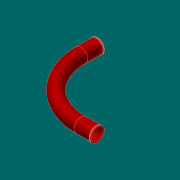
# Autodesk Inventor part: A1-19027-100-xx HCWI elbow
Saved by Autodesk Inventor 2017.3 (Build 213256000, 256)
## iProperties
Created: 2019-06-26
Part Number: A1-19027-100-xx HCWI elbow
Material: Iron, HCWI
Document SubType Name: Modeling
Designer: Graeme_Van_Dongen
Density: 7.33517 g/cm^3
Appearance: Iron Gray(1)
Mass: 7.05374e+06 g
Surface Area: 379961 cm^2
Volume: 961633 cm^3
Author: Graeme_Van_Dongen
Autodesk Inventor part; units mm, degrees
ref_plane "YZ Plane" through (0, 0, 0) normal (1, 0, 0) x (0, 1, 0)
ref_plane "XZ Plane" through (0, 0, 0) normal (0, 1, 0) x (-1, 0, 0)
ref_plane "XY Plane" through (0, 0, 0) normal (0, 0, 1) x (1, 0, 0)
sketch "Sketch1" plane through (0, 0, 0) normal (0, 0, 1) x (1, 0, 0)
  circle A0 centre (-3657.6, 0) radius 361.95
  circle A1 centre (-3657.6, 0) radius 412.75
  line L0 (0, -577.85) -> (0, 577.85) projected
  point P0 (0, 0)
  dimension "d0" = 723.9
  dimension "d1" = 825.5
  dimension "d2" = 3657.6
  constraints: 2 centre point, 1 coincident, 1 horizontal alignment
  measures "d0" diameter of A0
  measures "d1" diameter of A1
  measures "d2" distance of point (0, 0) A0.centre
revolve "Revolution1" add sketch "Sketch1" angle 90 about axis through (0, -10, 0) along (0, 1, 0)
sketch "Sketch2" plane through (-3657.6, 0, 0) normal (0, 0, -1) x (-1, 0, 0)
  circle A0 centre (0, 0) radius 361.95 projected
  circle A1 centre (0, 0) radius 412.75 projected
  point P0 (-3657.6, 0)
extrude "Extrusion1" add sketch "Sketch2" along normal blind 983.4
sketch "Sketch3" plane through (0, 0, 3657.6) normal (1, 0, 0) x (0, 0, -1)
  circle A0 centre (0, 0) radius 361.95 projected
  circle A1 centre (0, 0) radius 412.75 projected
  point P0 (3657.6, 0)
extrude "Extrusion2" add sketch "Sketch3" along normal blind 983.4
sketch "Sketch8" plane through (-3657.6, 0, -983.4) normal (0, 0, -1) x (-1, 0, 0)
  circle A0 centre (0, 0) radius 412.75 projected
  circle A1 centre (0, 0) radius 438.15
  point P0 (-3657.6, 0)
  dimension "d25" = 876.3
  constraints: 1 centre point, 1 coincident
  measures "d25" diameter of A1
extrude "Extrusion7" add sketch "Sketch8" against normal blind 50.8
sketch "Sketch9" plane through (983.4, 0, 3657.6) normal (1, 0, 0) x (0, 0, -1)
  circle A0 centre (0, 0) radius 412.75 projected
  circle A1 centre (0, 0) radius 361.95 projected
  circle A2 centre (0, 0) radius 438.15
  point P0 (3657.6, 0)
  dimension "d28" = 876.3
  constraints: 1 centre point, 1 coincident
  measures "d28" diameter of A2
extrude "Extrusion8" add sketch "Sketch9" against normal blind 50.8 contours A2
chamfer "Chamfer2" distance 25.4 angle 45 2 edges at (932.6, 0, 4070.35) (-3244.85, 0, -932.6)
sketch "Sketch5" plane through (-3657.6, 0, -983.4) normal (0, 0, -1) x (-1, 0, 0)
  circle A0 centre (0, 0) radius 434.721
  circle A1 centre (0, 0) radius 438.15 projected
  point P0 (-4064, 0)
  dimension "d11" = 869.442
  constraints: 1 centre point, 1 coincident
  measures "d11" diameter of A0
extrude "Extrusion4" cut sketch "Sketch5" against normal blind 25.4
sketch "Sketch7" plane through (983.4, 0, 3657.6) normal (1, 0, 0) x (0, 0, -1)
  circle A0 centre (0, 0) radius 434.721
  circle A1 centre (0, 0) radius 438.15 projected
  point P0 (4064, 0)
  dimension "d17" = 869.442
  constraints: 2 coincident, 1 centre point
  measures "d17" diameter of A0
extrude "Extrusion6" cut sketch "Sketch7" against normal blind 25.4
fillet "Fillet2" radius 0.7937 2 edges at (958, 0, 4092.321) (-3222.879, 0, -958)
equation "\"d6\" = d4"
equation "\"d28\" = d25"
equation "\"d29\" = d26"
equation "\"d31\" = -0.5 * d1 + 0.5 * d25"
equation "\"d17\" = d11"
equation "\"d18\" = d12"
equation "\"d4\" = 983.4"
equation "\"d26\" = 50.8"
equation "\"d12\" = 25.4"
body "Solid1"
